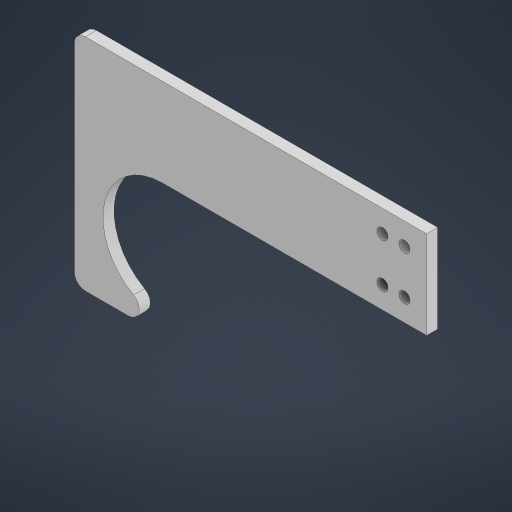
# Autodesk Inventor part: Climb_Hooks_2
Saved by Autodesk Inventor 2023 (Build 270158000, 158)
## iProperties
Created: 2024-02-21
Part Number: Climb_Hooks_2
Material: Generic
Document SubType Name: Modeling
Designer: kelle
Density: 1 g/cm^3
Appearance: Default
Author: kelle
Autodesk Inventor part; units mm, degrees
ref_plane "YZ Plane" through (0, 0, 0) normal (1, 0, 0) x (0, 1, 0)
ref_plane "XZ Plane" through (0, 0, 0) normal (0, 1, 0) x (-1, 0, 0)
ref_plane "XY Plane" through (0, 0, 0) normal (0, 0, 1) x (1, 0, 0)
sketch "Sketch1" plane through (0, 0, 0) normal (0, 0, 1) x (1, 0, 0)
  line L0 (38.1, -12.7) -> (-38.1, -12.7)
  line L1 (-38.1, -12.7) -> (-38.1, 12.7)
  line L2 (-38.1, 12.7) -> (38.1, 12.7)
  line L3 (38.1, 12.7) -> (38.1, -12.7)
  line L4 (38.1, -12.7) -> (-38.1, 12.7) construction
  line L5 (-38.1, -12.7) -> (38.1, 12.7) construction
  circle A0 centre (31.75, 6.35) radius 1.5875
  circle A1 centre (31.75, -6.35) radius 1.5875
  circle A2 centre (25.4, 6.35) radius 1.5875
  circle A3 centre (25.4, -6.35) radius 1.5875
  line L6 (-38.1, 12.7) -> (-63.5, 12.7)
  line L7 (-63.5, 12.7) -> (-63.5, -50.8)
  line L8 (-63.5, -50.8) -> (-38.1, -50.8)
  line L9 (-38.1, -50.8) -> (-38.1, 12.7)
  circle A4 centre (-38.1, -29.845) radius 17.145
  point P0 (0, 0)
  point P1 (-38.1, -46.99)
  dimension "d0" = 76.2
  dimension "d1" = 25.4
  dimension "d2" = 3.175
  dimension "d3" = 6.35
  dimension "d4" = 6.35
  dimension "d5" = 3.175
  dimension "d6" = 6.35
  dimension "d7" = 6.35
  dimension "d8" = 3.175
  dimension "d9" = 6.35
  dimension "d10" = 6.35
  dimension "d13" = 3.175
  dimension "d14" = 6.35
  dimension "d15" = 6.35
  dimension "d16" = 25.4
  dimension "d17" = 63.5
  dimension "d18" = 34.29
  dimension "d19" = 17.145
  constraints: 20 end point, 5 centre point, 4 parallel, 2 horizontal, 2 midpoint, 2 perpendicular, 1 point on line
  measures "d0" distance of L1.end L2.end
  measures "d1" distance of L0.end L1.end
  measures "d2" diameter of A0
  measures "d3" distance from line of L2 A0.centre
  measures "d4" distance from line of L3 A0.centre
  measures "d5" diameter of A1
  measures "d6" distance from line of L3 A1.centre
  measures "d7" distance from line of L0 A1.centre
  measures "d8" diameter of A2
  measures "d9" distance of A0.centre A2.centre
  measures "d10" distance from line of L2 A2.centre
  measures "d13" diameter of A3
  measures "d14" distance of A1.centre A3.centre
  measures "d15" distance from line of L0 A3.centre
  measures "d16" distance of L8.end L7.end
  measures "d17" distance of L7.end L6.end
  measures "d18" diameter of A4
  measures "d19" distance from line of L0 A4.centre
extrude "Extrusion1" add sketch "Sketch1" along normal blind 3.175 contours L0 L1 L2 L3 | A4 L9 L8 L7 L6 L1
fillet "Fillet1" radius 3.175 4 edges at (-38.1, -50.8, 1.5875) (-38.1, -46.99, 1.5875) (-63.5, -50.8, 1.5875) (-63.5, 12.7, 1.5875)
body "Solid1"
